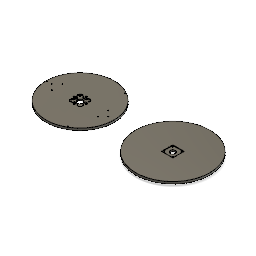
CNC Lazy Susan Bearing Wood Pieces (Autodesk Fusion 360 design; units mm, degrees)
Autodesk Fusion 360 part; units mm, degrees
sketch "Sketch1" plane through (0, 0, 0) normal (0, 1, 0) x (1, 0, 0)
  circle A0 centre (0, 0) radius 183.5
  circle A1 centre (0, 0) radius 177.5 construction
  circle A2 centre (-177.5, 0) radius 2
  circle A3 centre (88.75, -153.7195) radius 2
  circle A4 centre (88.75, 153.7195) radius 2
  circle A5 centre (0, 0) radius 15
  circle A6 centre (-24.5659, -24.5659) radius 1.95
  line L0 (22.5, -7.87) -> (22.5, 7.87)
  line L1 (-22.5, 7.87) -> (-22.5, -7.87)
  circle A7 centre (24.5659, 24.5659) radius 1.95
  arc A8 (7.87, -22.5) -> (22.5, -7.87) centre (20.1464, -20.1464) ccw
  arc A9 (22.5, 7.87) -> (7.87, 22.5) centre (20.1464, 20.1464) ccw
  line L2 (7.87, 22.5) -> (-7.87, 22.5)
  circle A10 centre (24.5659, -24.5659) radius 1.95
  arc A11 (-7.87, 22.5) -> (-22.5, 7.87) centre (-20.1464, 20.1464) ccw
  line L3 (-7.87, -22.5) -> (7.87, -22.5)
  arc A12 (-22.5, -7.87) -> (-7.87, -22.5) centre (-20.1464, -20.1464) ccw
  circle A13 centre (-24.5659, 24.5659) radius 1.95
  line L4 (22.55, -7.8288) -> (22.55, 7.8288)
  arc A14 (22.55, 7.8288) -> (7.8288, 22.55) centre (20.1464, 20.1464) ccw
  line L5 (7.8288, 22.55) -> (-7.8288, 22.55)
  arc A15 (-7.8288, 22.55) -> (-22.55, 7.8288) centre (-20.1464, 20.1464) ccw
  line L6 (-22.55, 7.8288) -> (-22.55, -7.8288)
  arc A16 (-22.55, -7.8288) -> (-7.8288, -22.55) centre (-20.1464, -20.1464) ccw
  line L7 (-7.8288, -22.55) -> (7.8288, -22.55)
  arc A17 (7.8288, -22.55) -> (22.55, -7.8288) centre (20.1464, -20.1464) ccw
  line L8 (0, -42.4264) -> (0, 42.4264) construction
  circle A18 centre (0, -32.4264) radius 1.95
  line L9 (42.4264, 0) -> (0, -42.4264)
  line L10 (0, -42.4264) -> (-42.4264, 0)
  line L11 (-42.4264, 0) -> (42.4264, 0) construction
  line L12 (-42.4264, 0) -> (-32.4264, 0)
  line L13 (-42.4264, 0) -> (0, 42.4264)
  circle A19 centre (-32.4264, 0) radius 1.95
  circle A20 centre (0, 32.4264) radius 1.95
  line L14 (0, 42.4264) -> (42.4264, 0)
  circle A21 centre (32.4264, 0) radius 1.95
  circle A22 centre (0, -32.4264) radius 4.45
  circle A23 centre (32.4264, 0) radius 4.45
  circle A24 centre (0, 32.4264) radius 4.45
  circle A25 centre (-32.4264, 0) radius 4.45
  line L15 (0, 0) -> (-152.4, 0) construction
  line L16 (-152.4, 0) -> (-124.1157, 28.2843) construction
  line L17 (-152.4, 0) -> (-99.7, 0) construction
  line L18 (-152.4, 0) -> (-124.1157, -28.2843) construction
  line L19 (-152.4, 0) -> (-99.7, 0) construction
  circle A26 centre (-152.4, 0) radius 1.95
  circle A27 centre (-124.1157, 28.2843) radius 1.95
  circle A28 centre (-124.1157, -28.2843) radius 1.95
  circle A29 centre (152.4, 0) radius 1.95
  circle A30 centre (124.1157, -28.2843) radius 1.95
  circle A31 centre (124.1157, 28.2843) radius 1.95
  dimension "d1" = 367
  dimension "d2" = 355
  dimension "d3" = 4
  dimension "d5" = 360
  dimension "d58" = 30
  dimension "d33" = 0.05
  dimension "d27" = 50
  dimension "d28" = 50
  dimension "d29" = 10.6775
  dimension "d55" = 60
  dimension "d56" = 60
  dimension "d57" = 10
  dimension "d59" = 3.9
  dimension "d60" = 2.5
  dimension "d61" = 2.5
  dimension "d62" = 2.5
  dimension "d63" = 2.5
  dimension "d65" = 45
  dimension "d66" = 40
  dimension "d67" = 45
  dimension "d68" = 40
  dimension "d69" = 3.9
  dimension "d70" = 3.9
  dimension "d71" = 3.9
  dimension "d73" = 360
  constraint coincident A0.centre A1.centre
  constraint concentric A0 A1
  constraint coincident A1 A2.centre
  constraint perpendicular L10 L13
  constraint parallel L10 L14
  constraint parallel L9 L13
  constraint parallel L11 L12
  constraint coincident L12.end A19.centre
  constraint perpendicular L6 L15
  constraint horizontal L17
  constraint horizontal L19
  constraint coincident L15.end L16.start
  constraint coincident L16.end A27.centre
  constraint coincident L18.end A28.centre
  measures "d1" diameter of A0
  measures "d2" diameter of A1
  measures "d3" diameter of A2
  measures "d58" diameter of A5
  measures "d55" distance of L9.start L8.end
  measures "d56" distance of L10.end L8.end
  measures "d57" distance of L10.end L12.end
  measures "d59" diameter of A19
  measures "d65" angle of L16 L17
  measures "d66" distance of L15.end L16.end
  measures "d67" angle of L18 L19
  measures "d68" distance of L15.end L18.end
  measures "d69" diameter of A26
  measures "d70" diameter of A27
  measures "d71" diameter of A28
extrude "Extrude1" add sketch "Sketch1" along normal blind 12.065 contours A0 | A5 | A6 | L0 L1 A8 A9 L2 A11 L3 A12 L9 L10 L13 L14 | L0 A8 A9 L4 A14 A17 L9 L14 | A8 A17 L9 | A8 L9 | A9 L14 | A9 A14 L14 | A8 L3 A12 A16 L7 A17 L9 L10 | L4 A14 A17 L9 L14 | A9 L2 A11 A14 L5 A15 L13 L14 | A16 L7 A17 L9 L10 | A14 L5 A15 L13 L14 | A12 A16 L10 | A12 L10 | A11 L13 | A11 A15 L13 | L1 A11 A12 A15 L6 A16 L10 L13 | A15 L6 A16 L10 L13 | A7 | A10 | A13 | A18 | A19 | A20 | A21 | A22 | A23 | A24 | A25 | A26 | A27 | A28 | A29 | A30 | A31 makes body 1
extrude "Extrude2" cut sketch "Sketch1" along normal up to surface (5 mm away) from surface at 7.065 contours A6 | L0 L1 A8 A9 L2 A11 L3 A12 L9 L10 L13 L14 | L0 A8 A9 L4 A14 A17 L9 L14 | A8 A17 L9 | A8 L9 | A9 L14 | A9 A14 L14 | A8 L3 A12 A16 L7 A17 L9 L10 | A9 L2 A11 A14 L5 A15 L13 L14 | A12 A16 L10 | A12 L10 | A11 L13 | A11 A15 L13 | L1 A11 A12 A15 L6 A16 L10 L13 | A7 | A10 | A13 bodies 1
extrude "Extrude3" cut sketch "Sketch1" along normal up to surface (12.065 mm away) contours A5 | A6 | A7 | A10 | A13 | A18 | A19 | A20 | A21 | A22 | A23 | A24 | A25 | A26 | A27 | A28 | A29 | A30 | A31 bodies 1
sketch "Sketch2" plane through (0, 12.065, 0) normal (0, 1, 0) x (-1, 0, 0)
  circle A0 centre (-88.75, -153.7195) radius 2
  circle A1 centre (177.5, 0) radius 2
  circle A2 centre (-88.75, 153.7195) radius 2
  circle A3 centre (0, 0) radius 183.5
  circle A4 centre (-500, 0) radius 200
  line L0 (7.8288, -22.55) -> (-7.8288, -22.55)
  arc A5 (-22.55, -7.8288) -> (-7.8288, -22.55) centre (-20.1464, -20.1464) ccw
  line L1 (-22.55, -7.8288) -> (-22.55, 7.8288)
  arc A6 (-7.8288, 22.55) -> (-22.55, 7.8288) centre (-20.1464, 20.1464) ccw
  line L2 (-7.8288, 22.55) -> (7.8288, 22.55)
  arc A7 (22.55, 7.8288) -> (7.8288, 22.55) centre (20.1464, 20.1464) ccw
  line L3 (22.55, 7.8288) -> (22.55, -7.8288)
  arc A8 (7.8288, -22.55) -> (22.55, -7.8288) centre (20.1464, -20.1464) ccw
  circle A9 centre (-500, -10) radius 1.25
  circle A10 centre (-490.4894, -3.0902) radius 1.25
  circle A11 centre (-509.5106, -3.0902) radius 1.25
  circle A12 centre (-505.8779, 8.0902) radius 2
  circle A13 centre (-490.4894, -3.0902) radius 2
  circle A14 centre (-494.1221, 8.0902) radius 1.25
  circle A15 centre (-494.1221, 8.0902) radius 2
  circle A16 centre (-500, -10) radius 2
  circle A17 centre (-494.1221, 8.0902) radius 1.25
  circle A18 centre (-505.8779, 8.0902) radius 1.25
  circle A19 centre (-509.5106, -3.0902) radius 2
  circle A20 centre (-505.8779, 8.0902) radius 1.25
  circle A21 centre (-490.4894, -3.0902) radius 1.25
  circle A22 centre (-500, 0) radius 14
  circle A23 centre (-500, -10) radius 1.25
  circle A24 centre (-500, 0) radius 14
  circle A25 centre (-509.5106, -3.0902) radius 1.25
  line L4 (-470, -30) -> (-530, 30) construction
  circle A26 centre (-477.0711, -22.9289) radius 1.95
  line L5 (-470, 30) -> (-470, -30)
  line L6 (-470, -30) -> (-530, -30)
  line L7 (-530, -30) -> (-470, 30) construction
  line L8 (-530, -30) -> (-522.9289, -22.9289)
  line L9 (-530, -30) -> (-530, 30)
  circle A27 centre (-522.9289, -22.9289) radius 1.95
  circle A28 centre (-522.9289, 22.9289) radius 1.95
  line L10 (-530, 30) -> (-470, 30)
  circle A29 centre (-477.0711, 22.9289) radius 1.95
  line L11 (-530.05, -30.05) -> (-530.05, 30.05)
  line L12 (-530.05, 30.05) -> (-469.95, 30.05)
  line L13 (-469.95, 30.05) -> (-469.95, -30.05)
  line L14 (-469.95, -30.05) -> (-530.05, -30.05)
  circle A30 centre (-32.4264, 0) radius 4.45
  circle A31 centre (0, 32.4264) radius 4.45
  circle A32 centre (0, -32.4264) radius 4.45
  circle A33 centre (32.4264, 0) radius 4.45
  circle A34 centre (124.1157, 28.2843) radius 1.95
  circle A35 centre (-124.1157, -28.2843) radius 1.95
  circle A36 centre (152.4, 0) radius 1.95
  circle A37 centre (-124.1157, 28.2843) radius 1.95
  circle A38 centre (-152.4, 0) radius 1.95
  circle A39 centre (124.1157, -28.2843) radius 1.95
  circle A40 centre (-500, 0) radius 192
  circle A41 centre (-308, 0) radius 2
  circle A42 centre (-404, 166.2769) radius 2
  circle A43 centre (-596, 166.2769) radius 2
  circle A44 centre (-692, 0) radius 2
  circle A45 centre (-596, -166.2769) radius 2
  circle A46 centre (-404, -166.2769) radius 2
  circle A47 centre (-500, 0) radius 185
  circle A48 centre (-500, 0) radius 167
  point P0 (-500, 0)
  point P1 (-500, 0)
  point P2 (-500, 0)
  point P3 (-500, 0)
  dimension "d34" = -0.75
  dimension "d35" = -0.75
  dimension "d15" = 0.75
  dimension "d16" = -0.75
  dimension "d38" = 0.75
  dimension "d50" = 60
  dimension "d51" = 60
  dimension "d52" = 10
  dimension "d36" = 3.9
  dimension "d54" = -0.05
  dimension "d74" = 400
  dimension "d76" = 384
  dimension "d77" = 4
  dimension "d80" = 360
  dimension "d81" = -15
  dimension "d82" = -33
  constraint coincident P3 P2
  constraint horizontal L6
  constraint perpendicular L6 L9
  constraint parallel L6 L10
  constraint parallel L5 L9
  constraint parallel L7 L8
  constraint coincident L8.end A27.centre
  constraint coincident A40 A41.centre
  measures "d50" distance of L5.start L4.end
  measures "d51" distance of L6.end L4.end
  measures "d52" distance of L6.end L8.end
  measures "d36" diameter of A27
  measures "d74" diameter of A4
  measures "d76" diameter of A40
  measures "d77" diameter of A41
extrude "Extrude4" add sketch "Sketch2" along normal blind 12.065 separate body contours A4 | A9 A23 | A10 A21 | A11 A25 | A12 | A13 | A14 A17 | A15 | A16 | A18 A20 | A19 | A22 A24 | A26 | L5 L6 L9 L10 | A27 | A28 | A29 | L11 L12 L13 L14 | A40 A41 | A40 A41 | A40 A41 A42 A43 A44 A45 A46 | A40 A42 | A40 A42 | A40 A46 | A40 A46 | A40 A43 | A40 A43 | A40 A45 | A40 A45 | A40 A44 | A40 A44 | A47 | A48 makes body 2
extrude "Extrude5" cut sketch "Sketch2" against normal blind 3 from surface at 12.065 contours A9 A23 | A10 A21 | A11 A25 | A12 | A13 | A14 A17 | A15 | A16 | A18 A20 | A19 | A22 A24 | L5 L6 L9 L10 | L11 L12 L13 L14 bodies 2
extrude "Extrude6" cut sketch "Sketch2" along normal up to surface (12.065 mm away) contours A9 A23 | A10 A21 | A11 A25 | A12 | A13 | A14 A17 | A15 | A16 | A18 A20 | A19 | A22 A24 | A26 | A27 | A28 | A29 bodies 2
equation "d10 = 5 mm + ( 7.065 mm - 5 mm )"
equation "d29 = 21.355 mm / 2"
